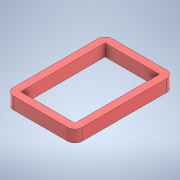
# Autodesk Inventor part: bumper simple
Saved by Autodesk Inventor 2022 (Build 260153000, 153)
## iProperties
Created: 2023-01-11
Part Number: bumper simple
Material: Generic
Document SubType Name: Modeling
Designer: s135320
Density: 1 g/cm^3
Appearance: Default
Author: s135320
Autodesk Inventor part; units mm, degrees
ref_plane "YZ Plane" through (0, 0, 0) normal (1, 0, 0) x (0, 1, 0)
ref_plane "XZ Plane" through (0, 0, 0) normal (0, 1, 0) x (-1, 0, 0)
ref_plane "XY Plane" through (0, 0, 0) normal (0, 0, 1) x (1, 0, 0)
sketch "Sketch1" plane through (0, 0, 0) normal (0, 1, 0) x (-1, 0, 0)
  line L0 (0, 0) -> (571.5, 0)
  line L1 (571.5, 0) -> (571.5, -889)
  line L2 (571.5, -889) -> (0, -889)
  line L3 (0, -889) -> (0, 0)
  line L4 (-76.2, 76.2) -> (647.7, 76.2)
  line L5 (647.7, 76.2) -> (647.7, -965.2)
  line L6 (647.7, -965.2) -> (-76.2, -965.2)
  line L7 (-76.2, -965.2) -> (-76.2, 76.2)
  dimension "d0" = 571.5
  dimension "d1" = 889
  dimension "d2" = 76.2
  dimension "d3" = 76.2
  dimension "d4" = 76.2
  dimension "d5" = 76.2
  constraints: 16 end point, 4 parallel, 2 horizontal, 2 perpendicular
  measures "d0" distance of L1.end L2.end
  measures "d1" distance of L2.end L0.start
  measures "d2" distance between parallel lines of L5 L1
  measures "d3" distance between parallel lines of L6 L2
  measures "d4" distance between parallel lines of L7 L3
  measures "d5" distance between parallel lines of L0 L4
extrude "Extrusion1" add sketch "Sketch1" along normal blind 127
fillet "Fillet1" radius 76.2 4 edges at (-647.7, 63.5, 76.2) (76.2, 63.5, 76.2) (76.2, 63.5, -965.2) (-647.7, 63.5, -965.2)
body "Solid1"
